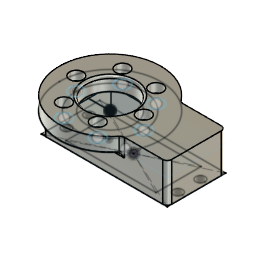
20Kg Servo Bracket v6 (Autodesk Fusion 360 design; units mm, degrees)
Autodesk Fusion 360 part; units mm, degrees
sketch "Sketch1" plane through (0, 0, 0) normal (0, 0, 1) x (1, 0, 0)
  line L0 (20, -10) -> (-20, -10)
  line L1 (-20, -10) -> (-20, 10)
  line L2 (-20, 10) -> (20, 10)
  line L3 (20, 10) -> (20, -10)
  line L4 (20, -10) -> (-20, 10) construction
  line L5 (-20, -10) -> (20, 10) construction
  line L6 (28, -13) -> (-28, -13)
  line L7 (-28, -13) -> (-28, 13)
  line L8 (-28, 13) -> (28, 13)
  line L9 (28, 13) -> (28, -13)
  line L10 (28, -13) -> (-28, 13) construction
  line L11 (-28, -13) -> (28, 13) construction
  circle A0 centre (-24.75, 5) radius 2
  line L12 (0, 0) -> (0, 3) construction
  line L13 (0, 3) -> (0, 0) construction
  line L14 (0, 0) -> (-3.4403, 0) construction
  circle A1 centre (-24.75, -5) radius 2
  circle A2 centre (24.75, 5) radius 2
  circle A3 centre (24.75, -5) radius 2
  line L15 (-20, 0) -> (-10.9, 0)
  dimension "d1" = 40
  dimension "d2" = 20
  dimension "d3" = 3
  dimension "d4" = 8
  dimension "d6" = 4
  dimension "d7" = 10
  dimension "d8" = 49.5
  dimension "d9" = 9.1
  constraint horizontal L0
  constraint perpendicular L0 L1
  constraint parallel L0 L2
  constraint parallel L1 L3
  constraint coincident L4 L12.start
  constraint coincident L5 L12.start
  constraint coincident L12.start L13.end
  constraint horizontal L6
  constraint perpendicular L6 L7
  constraint parallel L6 L8
  constraint parallel L7 L9
  constraint coincident L10 L12.start
  constraint coincident L11 L12.start
  constraint vertical L12
  constraint horizontal L14
  constraint symmetric A0 L14 A1
  constraint symmetric A0 L12 A2
  constraint symmetric L12 A1 A3
  constraint midpoint L1 L15.start
  constraint perpendicular L1 L15
  measures "d1" distance of L1.end L2.end
  measures "d2" distance of L0.end L1.end
  measures "d3" distance of L2 L8
  measures "d4" distance of L1 L7
  measures "d6" diameter of A0
  measures "d7" distance of A0.centre A1.centre
  measures "d8" distance of A1.centre A3.centre
  measures "d9" distance of L15.start L15.end
extrude "Extrude1" add sketch "Sketch1" along normal blind 11.25
sketch "Sketch2" plane through (0, 0, 11.25) normal (0, 0, 1) x (-1, 0, 0)
  circle A0 centre (-24.75, -5) radius 2
  circle A1 centre (-24.75, 5) radius 2
  line L0 (20, -10) -> (-20, -10)
  line L1 (-20, -10) -> (-20, 10)
  line L2 (-20, 10) -> (20, 10)
  line L3 (20, 10) -> (20, -10)
  circle A2 centre (24.75, 5) radius 2
  circle A3 centre (24.75, -5) radius 2
  line L4 (-28, -13) -> (28, -13)
  line L5 (28, -13) -> (28, 13)
  line L6 (28, 13) -> (-28, 13)
  line L7 (-28, 13) -> (-28, -13)
  line L8 (20, 0) -> (10.4, 0)
  circle A4 centre (10.4, 0) radius 15
  circle A5 centre (10.4, 0) radius 10.5
  circle A6 centre (10.4, 0) radius 22.5
  circle A7 centre (25.4, 0) radius 3
  circle A8 centre (17.9, 12.9904) radius 3
  circle A9 centre (2.9, 12.9904) radius 3
  circle A10 centre (-4.6, 0) radius 3
  circle A11 centre (2.9, -12.9904) radius 3
  circle A12 centre (17.9, -12.9904) radius 3
  dimension "d12" = 9.6
  dimension "d13" = 30
  dimension "d14" = 21
  dimension "d15" = 45
  dimension "d19" = 6
  dimension "d21" = 360
  constraint midpoint L3 L8.start
  constraint perpendicular L3 L8
  constraint coincident L8.end A4.centre
  constraint concentric A4 A5
  constraint concentric A5 A6
  constraint coincident A4 A7.centre
  measures "d12" distance of L8.start L8.end
  measures "d13" diameter of A4
  measures "d14" diameter of A5
  measures "d15" diameter of A6
  measures "d19" diameter of A7
extrude "Extrude2" add sketch "Sketch2" along normal blind 4 contours L0 L2 L3 A2 A3 A4 A5 A7 A8 A12 | L0 L3 A5 A12 | L0 L4 A5 A11 A12 | A3 L4 L5 A4 A7 A12 | L4 A4 A11 A12 | A3 A4 | A3 A4 | L2 L3 A5 A8 | L0 L2 A4 A5 A9 A10 A11 | L4 L5 L6 A4 A6 A7 A8 A9 A11 A12 | L2 L6 A5 A8 A9 | L0 A4 A11 | L0 L4 A4 A6 A11 | A2 L5 L6 A4 A7 A8 | L6 A4 A8 A9 | L0 L2 A4 A6 A10 | L2 A4 A9 | A2 A4 | A2 A4 | L2 L6 A4 A6 A9
extrude "Extrude3" add sketch "Sketch2" along normal blind 2 contours L0 L4 A4 A12 | L0 A12 | L4 A4 A12 | L4 A4 A12 | L4 A4 A12 | L4 A4 A11 | L0 L4 A4 A11 | L0 A11 | L4 A4 A11 | L4 A4 A11 | A4 A7 | L5 A4 A7 | L2 A8 | L2 L6 A4 A8 | L2 A9 | L2 L6 A4 A9 | L5 A7 | L6 A4 A8 | L6 A4 A8 | L6 A4 A8 | L6 A4 A9 | A4 A10 | A4 A10 | L6 A4 A9 | L6 A4 A9
extrude "Extrude5" add sketch "Sketch2" along normal blind 4 contours A0 | A1 | L0 L1 L2 L4 L6 L7 A6 | L0 L1 L2 A6
fillet "Fillet1" radius 2 7 edges at (7.9644, 13, 13.25) (-10.0178, 13, 11.25) (-28, 13, 5.625) (-28, 0, 11.25) (-28, -13, 5.625) (-10.0178, -13, 11.25) (7.9644, -13, 13.25)
fillet "Fillet2" radius 2 2 edges at (28, 13, 7.625) (28, -13, 7.625)
sketch "Sketch3" plane through (0, 0, 15.25) normal (0, 0, 1) x (-1, 0, 0)
  arc A0 (-26, 13) -> (-28, 11) centre (-26, 11) ccw
  line L0 (-28, 11) -> (-28, -11)
  arc A1 (-28, -11) -> (-26, -13) centre (-26, -11) ccw
  line L1 (-26, -13) -> (-8.9714, -13)
  arc A2 (-7.39, -13.7755) -> (-8.9714, -13) centre (-8.9714, -15) ccw
  arc A3 (-7.39, -13.7755) -> (-7.39, 13.7755) centre (10.4, 0) ccw
  arc A4 (-8.9714, 13) -> (-7.39, 13.7755) centre (-8.9714, 15) ccw
  line L2 (-8.9714, 13) -> (-26, 13)
  circle A5 centre (2.9, -12.9904) radius 3
  circle A6 centre (17.9, 12.9904) radius 3
  circle A7 centre (2.9, 12.9904) radius 3
  circle A8 centre (17.9, -12.9904) radius 3
  circle A9 centre (-4.6, 0) radius 3
  circle A10 centre (25.4, 0) radius 3
  circle A11 centre (10.4, 0) radius 10.5
  circle A12 centre (10.4, 0) radius 22.5
  circle A13 centre (17.9, -12.9904) radius 3
  circle A14 centre (2.9, -12.9904) radius 3
  circle A15 centre (-4.6, 0) radius 3
  circle A16 centre (2.9, 12.9904) radius 3
  circle A17 centre (17.9, 12.9904) radius 3
  circle A18 centre (25.4, 0) radius 3
  constraint concentric A3 A12
  constraint concentric A8 A13
  constraint concentric A5 A14
  constraint concentric A9 A15
  constraint concentric A7 A16
  constraint concentric A6 A17
  constraint concentric A10 A18
extrude "Extrude6" add sketch "Sketch3" along normal blind 2
fillet "Fillet5" radius 1 1 edges at (-0.6106, -3.797, 17.25)
